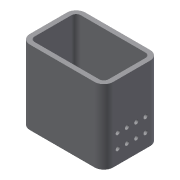
# Autodesk Inventor part: pullbox
Saved by Autodesk Inventor 2016 (Build 200138000, 138)
## iProperties
Created: 2014-12-12
Part Number: pullbox
Material: ABS Plastic
Document SubType Name: Modeling
Designer: Dave
Density: 1.06 g/cm^3
Appearance: Smooth - White
Author: Dave
Autodesk Inventor part; units mm, degrees
ref_plane "YZ Plane" through (0, 0, 0) normal (1, 0, 0) x (0, 1, 0)
ref_plane "XZ Plane" through (0, 0, 0) normal (0, 1, 0) x (-1, 0, 0)
ref_plane "XY Plane" through (0, 0, 0) normal (0, 0, 1) x (1, 0, 0)
sketch "Sketch1" plane through (0, 0, 0) normal (0, 1, 0) x (-1, 0, 0)
  line L0 (101.6, 0) -> (812.8, 0)
  line L1 (914.4, 101.6) -> (914.4, 508)
  line L2 (812.8, 609.6) -> (101.6, 609.6)
  line L3 (0, 508) -> (0, 101.6)
  arc A0 (101.6, 609.6) -> (0, 508) centre (101.6, 508) ccw
  arc A1 (0, 101.6) -> (101.6, 0) centre (101.6, 101.6) ccw
  arc A2 (812.8, 0) -> (914.4, 101.6) centre (812.8, 101.6) ccw
  arc A3 (914.4, 508) -> (812.8, 609.6) centre (812.8, 508) ccw
  point P0 (0, 0)
  point P1 (914.4, 609.6)
  point P2 (914.4, 0)
  point P3 (0, 609.6)
  dimension "d0" = 914.4
  dimension "d1" = 609.6
  dimension "d9" = 101.6
  constraints: 8 end point, 8 point on circle, 8 point on line, 8 tangent, 4 centre point, 3 equal radius, 2 parallel, 1 horizontal, 1 perpendicular
  measures "d0" distance of point (0, 609.6) point (914.4, 609.6)
  measures "d1" distance of point (914.4, 609.6) point (914.4, 0)
  measures "d9" radius of A0
extrude "Extrusion1" add sketch "Sketch1" along normal blind 50.8
sketch "Sketch3" plane through (0, 50.8, 0) normal (0, 1, 0) x (1, 0, 0)
  line L0 (0, -508) -> (0, -101.6) projected
  arc A0 (0, -101.6) -> (-101.6, 0) centre (-101.6, -101.6) ccw projected
  line L1 (-101.6, 0) -> (-812.8, 0) projected
  arc A1 (-812.8, 0) -> (-914.4, -101.6) centre (-812.8, -101.6) ccw projected
  line L2 (-914.4, -101.6) -> (-914.4, -508) projected
  arc A2 (-914.4, -508) -> (-812.8, -609.6) centre (-812.8, -508) ccw projected
  line L3 (-812.8, -609.6) -> (-101.6, -609.6) projected
  arc A3 (-101.6, -609.6) -> (0, -508) centre (-101.6, -508) ccw projected
  line L4 (-812.8, -50.8) -> (-101.6, -50.8)
  arc A4 (-50.8, -101.6) -> (-101.6, -50.8) centre (-101.6, -101.6) ccw
  line L5 (-50.8, -101.6) -> (-50.8, -508)
  arc A5 (-101.6, -558.8) -> (-50.8, -508) centre (-101.6, -508) ccw
  line L6 (-101.6, -558.8) -> (-812.8, -558.8)
  arc A6 (-863.6, -508) -> (-812.8, -558.8) centre (-812.8, -508) ccw
  line L7 (-863.6, -508) -> (-863.6, -101.6)
  arc A7 (-812.8, -50.8) -> (-863.6, -101.6) centre (-812.8, -101.6) ccw
  point P0 (0, 0)
  dimension "d10" = 50.8
  constraints: 8 end point, 8 point on circle, 4 centre point, 7 other
  measures "d10" distance between parallel lines of L4 L1
extrude "Extrusion3" add sketch "Sketch3" along normal blind 762
sketch "Sketch10" plane through (0, 0, 508) normal (1, 0, 0) x (0, 0, -1)
  circle A0 centre (50.8, 152.4) radius 22.5
  circle A1 centre (152.4, 152.4) radius 22.5
  circle A2 centre (254, 152.4) radius 22.5
  circle A3 centre (355.6, 152.4) radius 22.5
  line L0 (0, 0) -> (0, 812.8) projected
  line L1 (0, 0) -> (406.4, 0) projected
  circle A4 centre (50.8, 304.8) radius 22.5
  circle A5 centre (152.4, 304.8) radius 22.5
  circle A6 centre (254, 304.8) radius 22.5
  circle A7 centre (355.6, 304.8) radius 22.5
  dimension "d56" = 45
  dimension "d57" = 45
  dimension "d58" = 45
  dimension "d59" = 45
  dimension "d60" = 50.8
  dimension "d61" = 101.6
  dimension "d62" = 101.6
  dimension "d63" = 101.6
  dimension "d64" = 152.4
  dimension "d67" = 45
  dimension "d68" = 45
  dimension "d69" = 45
  dimension "d70" = 45
  dimension "d71" = 152.4
  constraints: 8 centre point, 6 horizontal alignment, 4 vertical alignment
  measures "d56" diameter of A0
  measures "d57" diameter of A1
  measures "d58" diameter of A2
  measures "d59" diameter of A3
  measures "d60" distance from line of A0.centre L0
  measures "d61" distance of A1.centre A0.centre
  measures "d62" distance of A2.centre A1.centre
  measures "d63" distance of A3.centre A2.centre
  measures "d64" distance from line of L1 A0.centre
  measures "d67" diameter of A4
  measures "d68" diameter of A5
  measures "d69" diameter of A6
  measures "d70" diameter of A7
  measures "d71" distance of A0.centre A4.centre
extrude "Extrusion4" cut sketch "Sketch10" against normal through all
body "Solid1"
